plug-sleeve-stub (Autodesk Fusion 360 design; units mm, degrees)
Autodesk Fusion 360 part; units mm, degrees
sketch "Sketch20" plane through (0, 0, 0) normal (0, 0, 1) x (1, 0, 0)
  line L0 (-44.25, -31.25) -> (44.25, -31.25)
  line L1 (44.25, -31.25) -> (44.25, 31.25)
  line L2 (44.25, 31.25) -> (-44.25, 31.25)
  line L3 (-44.25, 31.25) -> (-44.25, -31.25)
extrude "Extrude16" add sketch "Sketch20" along normal blind 8
fillet "Fillet3" radius 7 4 edges at (-44.25, 31.25, 4) (44.25, 31.25, 4) (44.25, -31.25, 4) (-44.25, -31.25, 4)
ref_plane "WorkPlane17" through (0, 0, 8) normal (0, 0, 1) x (1, 0, 0)
sketch "Sketch21" plane through (0, 0, 8) normal (0, 0, 1) x (1, 0, 0)
  line L0 (-34.25, -21.25) -> (34.25, -21.25)
  line L1 (34.25, -21.25) -> (34.25, 21.25)
  line L2 (34.25, 21.25) -> (-34.25, 21.25)
  line L3 (-34.25, 21.25) -> (-34.25, -21.25)
  line L4 (-31.25, -18.25) -> (31.25, -18.25)
  line L5 (31.25, -18.25) -> (31.25, 18.25)
  line L6 (31.25, 18.25) -> (-31.25, 18.25)
  line L7 (-31.25, 18.25) -> (-31.25, -18.25)
extrude "Extrude17" add sketch "Sketch21" along normal blind 30
fillet "Fillet4" radius 2.5 4 edges at (-34.25, 21.25, 23) (34.25, 21.25, 23) (34.25, -21.25, 23) (-34.25, -21.25, 23)
sketch "Sketch22" plane through (0, 0, 8) normal (0, 0, 1) x (1, 0, 0)
  line L0 (-44.25, -31.25) -> (44.25, -31.25)
  line L1 (44.25, -31.25) -> (44.25, 31.25)
  line L2 (44.25, 31.25) -> (-44.25, 31.25)
  line L3 (-44.25, 31.25) -> (-44.25, -31.25)
  line L4 (-39.25, -26.5) -> (39.25, -26.5)
  line L5 (39.25, -26.5) -> (39.25, 26.5)
  line L6 (39.25, 26.5) -> (-39.25, 26.5)
  line L7 (-39.25, 26.5) -> (-39.25, -26.5)
extrude "Extrude18" add sketch "Sketch22" along normal blind 25
sketch "Sketch23" plane through (0, 0, 8) normal (0, 0, 1) x (1, 0, 0)
  line L0 (-44.25, -31.25) -> (-39.25, -31.25)
  line L1 (-39.25, -31.25) -> (-39.25, 31.25)
  line L2 (-39.25, 31.25) -> (-44.25, 31.25)
  line L3 (-44.25, 31.25) -> (-44.25, -31.25)
extrude "Extrude19" cut sketch "Sketch23" along normal blind 25
fillet "Fillet5" radius 5 68 edges at (-33.5178, -20.5178, 8) (0, -21.25, 8) (33.5178, -20.5178, 8) (34.25, 0, 8) (33.5178, 20.5178, 8) (0, 21.25, 8) (-33.5178, 20.5178, 8) (-34.25, 0, 8) (0, -21.25, 8) (-33.5178, -20.5178, 8) (-34.25, 0, 8) (-33.5178, 20.5178, 8) (0, 21.25, 8) (33.5178, 20.5178, 8) (34.25, 0, 8) (33.5178, -20.5178, 8) (33.5178, -20.5178, 8) (34.25, 0, 8) (33.5178, 20.5178, 8) (0, 21.25, 8) (-33.5178, 20.5178, 8) (-34.25, 0, 8) (-33.5178, -20.5178, 8) (0, -21.25, 8) (33.5178, 20.5178, 8) (0, 21.25, 8) (-33.5178, 20.5178, 8) (-34.25, 0, 8) (-33.5178, -20.5178, 8) (0, -21.25, 8) (33.5178, -20.5178, 8) (34.25, 0, 8) (0, 21.25, 8) (33.5178, 20.5178, 8) (34.25, 0, 8) (33.5178, -20.5178, 8) (0, -21.25, 8) (-33.5178, -20.5178, 8) (-34.25, 0, 8) (-33.5178, 20.5178, 8) (-33.5178, 20.5178, 8) (-34.25, 0, 8) (-33.5178, -20.5178, 8) (0, -21.25, 8) (33.5178, -20.5178, 8) (34.25, 0, 8) (33.5178, 20.5178, 8) (0, 21.25, 8) (-34.25, 0, 8) (-33.5178, 20.5178, 8) (0, 21.25, 8) (33.5178, 20.5178, 8) (34.25, 0, 8) (33.5178, -20.5178, 8) (0, -21.25, 8) (-33.5178, -20.5178, 8) (0, -18.25, 8) (31.25, 0, 8) (0, 18.25, 8) (-31.25, 0, 8) (34.25, 0, 8) (33.5178, -20.5178, 8) (0, -21.25, 8) (-33.5178, -20.5178, 8) (-34.25, 0, 8) (-33.5178, 20.5178, 8) (0, 21.25, 8) (33.5178, 20.5178, 8)
named bodies: "plug_sleeve_stub"
